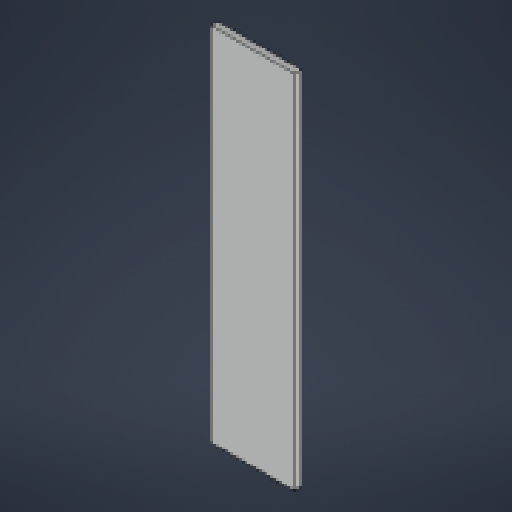
# Autodesk Inventor part: PLATE,BOTTOM
Saved by Autodesk Inventor 2026.1 (Build 301233020, 233B)
## iProperties
Created: 2026-03-19
Part Number: PLATE,BOTTOM
Material: Aluminum 6061
Document SubType Name: Sheet Metal
Designer: Owen L
Mass: 276.532 g
Surface Area: 362.902 cm^2
Volume: 102.419 cm^3
Density: 2.7 g/cm^3
Sheet Metal Rule: Default
Appearance: Aluminum - Flat
Author: Owen L
Autodesk Inventor part; units mm, degrees
ref_plane "YZ Plane" through (0, 0, 0) normal (1, 0, 0) x (0, 1, 0)
ref_plane "XZ Plane" through (0, 0, 0) normal (0, 1, 0) x (-1, 0, 0)
ref_plane "XY Plane" through (0, 0, 0) normal (0, 0, 1) x (1, 0, 0)
sketch "Sketch1" plane through (0, 0, 0) normal (0, 0, 1) x (1, 0, 0)
  line L0 (31.75, -127) -> (-31.75, -127)
  line L1 (-31.75, -127) -> (-31.75, 127)
  line L2 (-31.75, 127) -> (31.75, 127)
  line L3 (31.75, 127) -> (31.75, -127)
  line L4 (31.75, -127) -> (-31.75, 127) construction
  line L5 (-31.75, -127) -> (31.75, 127) construction
  point P0 (0, 0)
  dimension "d0" = 254
  dimension "d1" = 63.5
  measures "d0" distance of L0.end L1.end
  measures "d1" distance of L0.start L0.end
extrude "Plate1" add sketch "Sketch1" along normal blind 6.35
equation "\"d2\" = Thickness"
equation "\"BendRadius\" = Thickness"
equation "\"BendReliefWidth\" = Thickness"
equation "\"BendReliefDepth\" = 0.5 * Thickness"
equation "\"CornerReliefSize\" = 4 * Thickness"
equation "\"MinimumRemnant\" = 2 * Thickness"
equation "\"TransitionRadius\" = BendRadius"
equation "\"JacobiRadiusSize\" = BendRadius"
equation "\"GapSize\" = Thickness"
equation "\"Thickness\" = 6.35"
body "Solid1"
